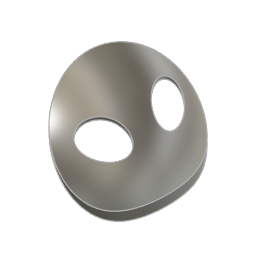
cara (Autodesk Fusion 360 design; units mm, degrees)
part number: 2026-06-26-00-47-44-738
Autodesk Fusion 360 part; units mm, degrees
note: some values were not read from the file. Set by a fixed rule: which face or edge a step refers to.
sketch "Boceto1" plane through (0, 0, 0) normal (0, 1, 0) x (1, 0, 0)
  arc A0 (0, -57.5) -> (0, 57.5) centre (0, 0) ccw
  line L0 (0, 0) -> (0, 57.5)
  arc A1 (0, -56.5) -> (0, 56.5) centre (0, 0) ccw
  line L1 (0, 0) -> (0, -56.5)
  line L2 (0, -56.5) -> (0, -57.5)
  line L3 (56.5, 0) -> (55.5708, 0)
  ellipse E0 centre (37.1474, 0) end of major axis (37.1474, 31.9112) minor radius 18.4234
  line L4 (37.1474, -31.9112) -> (37.1474, 31.9112) construction
  line L5 (55.5708, 0) -> (18.724, 0) construction
  ellipse E1 centre (40.6799, 14.9999) end of major axis (35.6799, 23.6602) minor radius 5
  line L6 (45.6799, 6.3397) -> (35.6799, 23.6602) construction
  line L7 (45.01, 17.4999) -> (36.3498, 12.4999) construction
  line L8 (40.6799, 14.9999) -> (44.6474, 14.9999) construction
  ellipse E2 centre (40.7, -15) end of major axis (35.7, -23.6603) minor radius 5
  line L9 (45.7, -6.3397) -> (35.7, -23.6603) construction
  line L10 (36.3699, -12.5) -> (45.0301, -17.5) construction
  line L11 (40.7, -15) -> (44.6474, -15) construction
  point P0 (37.1474, 0)
  dimension "d2" = 57.5
  dimension "d3" = 56.5
  dimension "d4" = 19.3526
  dimension "d5" = 63.8224
  dimension "d6" = 36.8469
  dimension "d10" = 20
  dimension "d11" = 120
  dimension "d12" = 10
  dimension "d13" = 20
  dimension "d14" = 120
  dimension "d15" = 10
  constraint coincident A0.centre L0.start
  constraint vertical L0
  constraint coincident L0 A1.start
  constraint parallel L1 L2
  constraint midpoint A1 L3.start
  constraint horizontal L3
  constraint coincident E0 L4.start
  constraint coincident E0 L4.end
  constraint coincident E0 L3.end
  constraint coincident E0 L5.end
  constraint perpendicular L3 L4
  constraint coincident P0 E0.centre
  constraint coincident E1 L6.start
  constraint coincident E1 L6.end
  constraint coincident E1 L7.start
  constraint coincident E1 L7.end
  constraint horizontal L8
  constraint coincident E2 L9.start
  constraint coincident E2 L9.end
  constraint coincident E2 L10.start
  constraint coincident E2 L10.end
  constraint horizontal L11
  measures "d2" radius of A0
  measures "d3" radius of A1
  measures "d4" distance of L3.start P0
  measures "d5" distance of E0
  measures "d10" distance of E1
  measures "d11" angle of L6 L8
  measures "d12" distance of E1
  measures "d13" distance of E2
  measures "d14" angle of L9 L11
  measures "d15" distance of E2
revolve "Revolución1" add sketch "Boceto1" angle 90 about axis through (0, 0, 0) along (0, 0, 1) contours A0 L0 A1 L2 makes body 1
extrude "Extruir1" cut sketch "Boceto1" along normal blind 72 contours E0 | E1 | E2 keep common part bodies 1
delete_face "SuprimirCaras1" 1 faces at (55.3505, 13.2646, 4.9207) on bodies 1
delete_face "SuprimirCaras2" 2 faces at (54.5143, 13.5919, 12.2352) (53.5662, 13.3556, 12.0225) on bodies 1
revolve "Revolución2" add sketch "Boceto1" angle 90 about axis through (0, 0, 0) along (0, 0, 1) separate body contours A0 L0 A1 L2 makes body 2
extrude "Extruir2" cut sketch "Boceto1" along normal blind 60 contours E0 keep common part bodies 2
